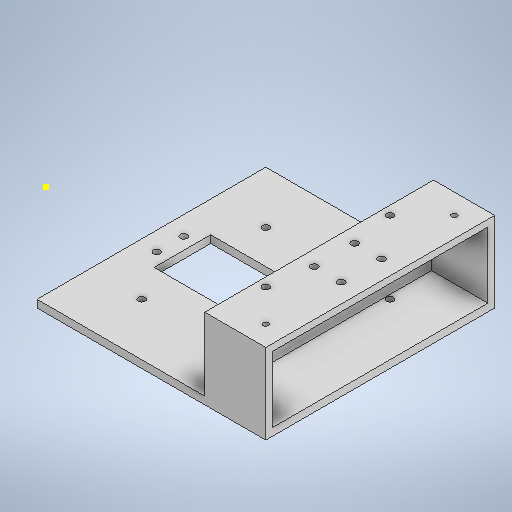
# Autodesk Inventor part: LowerHead
Saved by Autodesk Inventor 2025 (Build 290162000, 162)
## iProperties
Created: 2025-09-02
Part Number: LowerHead
Material: Generic
Document SubType Name: Modeling
Designer: wangb
Density: 1 g/cm^3
Appearance: Default
Author: wangb
Autodesk Inventor part; units mm, degrees
ref_plane "YZ Plane" through (0, 0, 0) normal (1, 0, 0) x (0, 1, 0)
ref_plane "XZ Plane" through (0, 0, 0) normal (0, 1, 0) x (-1, 0, 0)
ref_plane "XY Plane" through (0, 0, 0) normal (0, 0, 1) x (1, 0, 0)
sketch "Sketch1" plane through (0, 0, 0) normal (0, 1, 0) x (-1, 0, 0)
  line L0 (-7.3056, 10.788) -> (-92.3056, 10.788)
  line L1 (-92.3056, 10.788) -> (-92.3056, -74.212)
  line L2 (-92.3056, -74.212) -> (-7.3056, -74.212)
  line L3 (-7.3056, -74.212) -> (-7.3056, 10.788)
  line L4 (-18.8056, -21.212) -> (-59.8056, -21.212)
  line L5 (-59.8056, -21.212) -> (-59.8056, -42.212)
  line L6 (-59.8056, -42.212) -> (-18.8056, -42.212)
  line L7 (-18.8056, -42.212) -> (-18.8056, -21.212)
  circle A0 centre (-14.3056, -26.712) radius 1.3
  circle A1 centre (-14.3056, -36.712) radius 1.3
  circle A2 centre (-64.3056, -26.712) radius 1.3
  circle A3 centre (-64.3056, -36.712) radius 1.3
  circle A4 centre (-75.3056, -39.212) radius 1.3
  circle A5 centre (-85.3056, -39.212) radius 1.3
  circle A6 centre (-75.3056, -24.212) radius 1.3
  circle A7 centre (-85.3052, -24.1286) radius 1.3
  point P0 (0, 0)
  dimension "d0" = 85
  dimension "d1" = 85
  dimension "d2" = 41
  dimension "d3" = 21
  dimension "d4" = 32
  dimension "d5" = 11.5
  dimension "d6" = 2.6
  dimension "d7" = 2.6
  dimension "d8" = 10
  dimension "d9" = 5.5
  dimension "d10" = 5.5
  dimension "d11" = 2.6
  dimension "d12" = 2.6
  dimension "d13" = 10
  dimension "d14" = 5.5
  dimension "d15" = 50
  dimension "d16" = 50
  dimension "d17" = 4.5
  dimension "d31" = 2.6
  dimension "d32" = 2.6
  dimension "d33" = 10
  dimension "d34" = 2.6
  dimension "d35" = 2.6
  dimension "d36" = 10
  dimension "d37" = 15
  dimension "d38" = 35
  dimension "d39" = 17
  dimension "d40" = 17
  constraints: 16 end point, 8 centre point, 4 parallel, 2 horizontal, 2 perpendicular
  measures "d0" distance of L2.end L1.end
  measures "d1" distance of L1.end L0.end
  measures "d2" distance of L6.end L5.end
  measures "d3" distance of L5.end L4.end
  measures "d4" distance between parallel lines of L2 L6
  measures "d5" distance between parallel lines of L3 L7
  measures "d6" diameter of A0
  measures "d7" diameter of A1
  measures "d8" distance of A1.centre A0.centre
  measures "d9" vertical distance of L4.start A0.centre
  measures "d10" vertical distance of L6.end A1.centre
  measures "d11" diameter of A2
  measures "d12" diameter of A3
  measures "d13" distance of A3.centre A2.centre
  measures "d14" vertical distance of L5.end A3.centre
  measures "d15" distance of A2.centre A0.centre
  measures "d16" distance of A3.centre A1.centre
  measures "d17" distance from line of L5 A2.centre
  measures "d31" diameter of A4
  measures "d32" diameter of A5
  measures "d33" distance of A5.centre A4.centre
  measures "d34" diameter of A6
  measures "d35" diameter of A7
  measures "d36" distance of A7.centre A6.centre
  measures "d37" distance of A6.centre A4.centre
  measures "d38" distance from line of L2 A4.centre
  measures "d39" distance from line of A6.centre L1
  measures "d40" distance from line of L1 A4.centre
extrude "Extrusion1" add sketch "Sketch1" along normal blind 2.8 contours L3 L2 L1 L0 | A4 | A5 | A6 | A7
sketch "Sketch2" plane through (0, 2.8, 0) normal (0, 1, 0) x (1, 0, 0)
  line L0 (92.3056, -10.788) -> (92.3056, 74.212) projected
  line L1 (92.3056, 74.212) -> (7.3056, 74.212) projected
  line L2 (7.3056, -10.788) -> (92.3056, -10.788) projected
  point P0 (0, 0)
extrude "Extrusion2" [suppressed]
sketch "Sketch3" plane through (0, 2.8, 0) normal (0, 1, 0) x (1, 0, 0)
  line L0 (7.3056, -10.788) -> (92.3056, -10.788) projected
  line L1 (92.3056, 74.212) -> (7.3056, 74.212) projected
  line L2 (92.3056, -10.788) -> (69.6056, -10.788)
  line L3 (69.6056, -10.788) -> (69.6056, 74.212)
  line L4 (69.6056, 74.212) -> (92.3056, 74.212)
  line L5 (92.3056, 74.212) -> (92.3056, -10.788)
  circle A0 centre (64.3056, 36.712) radius 1.3 projected
  circle A1 centre (75.3056, 24.212) radius 1 projected
  circle A2 centre (75.3056, 24.212) radius 1
  circle A3 centre (75.3056, 39.212) radius 1 projected
  circle A4 centre (75.3056, 39.212) radius 1
  circle A5 centre (85.3056, 39.212) radius 1 projected
  circle A6 centre (85.3056, 39.212) radius 1
  circle A7 centre (85.3056, 24.212) radius 1 projected
  circle A8 centre (85.3056, 24.212) radius 1
  circle A9 centre (84.8056, 66.712) radius 0.95 projected
  circle A10 centre (84.8056, 66.712) radius 1
  circle A11 centre (84.8056, -3.288) radius 0.95 projected
  circle A12 centre (84.8056, -3.288) radius 1
  point P0 (0, 0)
  dimension "d55" = 4
  dimension "d56" = 2
  dimension "d57" = 2
  constraints: 8 end point, 6 centre point, 6 coincident, 2 parallel, 1 horizontal, 1 perpendicular, 1 point on line
  measures "d55" distance edge to line of A0 L3
  measures "d56" diameter of A10
  measures "d57" diameter of A12
extrude "Extrusion3" add sketch "Sketch3" along normal blind 27 contours L3 L1 L5 L0
sketch "Sketch4" plane through (92.3056, 0, 10.788) normal (1, 0, 0) x (0, 0, -1)
  line L0 (85, 2.8) -> (0, 2.8) projected
  line L1 (2.5, 27.3) -> (82.5, 27.3)
  line L2 (82.5, 27.3) -> (82.5, 2.8)
  line L3 (82.5, 2.8) -> (2.5, 2.8)
  line L4 (2.5, 2.8) -> (2.5, 27.3)
  line L5 (0, 0) -> (0, 29.8) projected
  line L6 (85, 0) -> (85, 29.8) projected
  line L7 (0, 0) -> (85, 0) projected
  line L8 (0, 29.8) -> (85, 29.8) projected
  point P0 (10.788, 0)
  point P1 (2.5, 2.8)
  dimension "d60" = 2.5
  dimension "d61" = 2.5
  dimension "d62" = 2.8
  dimension "d63" = 2.5
  constraints: 8 end point, 2 parallel, 1 horizontal, 1 perpendicular, 1 point on line
  measures "d60" distance between parallel lines of L5 L4
  measures "d61" distance between parallel lines of L6 L2
  measures "d62" distance between parallel lines of L7 L0
  measures "d63" distance between parallel lines of L8 L1
extrude "Extrusion4" cut sketch "Sketch4" against normal blind 21 contours L0 L4 L1 L2
sketch "Sketch5" plane through (0, 0, 0) normal (0, -1, 0) x (1, 0, 0)
  circle A0 centre (26.7535, -8.6599) radius 1.3
  circle A1 centre (72.8576, -8.66) radius 1.3
  circle A2 centre (26.7536, -54.764) radius 1.3
  circle A3 centre (72.8576, -54.764) radius 1.3
  line L0 (7.3056, 10.788) -> (92.3056, 10.788) projected
  line L1 (92.3056, 10.788) -> (92.3056, -74.212) projected
  line L2 (7.3056, -74.212) -> (7.3056, 10.788) projected
  line L3 (92.3056, -74.212) -> (7.3056, -74.212) projected
  point P0 (0, 0)
  point P1 (49.2547, -32.4518)
  point P2 (49.2547, -32.4518)
  dimension "d66" = 2.6
  dimension "d67" = 2.6
  dimension "d68" = 2.6
  dimension "d69" = 2.6
  dimension "d70" = 46.1041
  dimension "d71" = 46.1041
  dimension "d72" = 46.1041
  dimension "d73" = 46.1041
  dimension "d74" = 19.448
  dimension "d75" = 19.448
  dimension "d76" = 19.448
  dimension "d77" = 19.448
  constraints: 4 centre point
  measures "d66" diameter of A0
  measures "d67" diameter of A1
  measures "d68" diameter of A2
  measures "d69" diameter of A3
  measures "d70" distance of A1.centre A0.centre
  measures "d71" distance of A2.centre A0.centre
  measures "d72" distance of A3.centre A1.centre
  measures "d73" distance of A3.centre A2.centre
  measures "d74" distance from line of L0 A1.centre
  measures "d75" distance from line of L1 A1.centre
  measures "d76" distance from line of L2 A2.centre
  measures "d77" distance from line of L3 A2.centre
extrude "Extrusion5" cut sketch "Sketch5" against normal blind 100 contours A0 | A1 | A2 | A3
sketch "Sketch6" plane through (0, 29.8, 0) normal (0, 1, 0) x (1, 0, 0)
  point P0 (0, 0)
sketch "Sketch7" plane through (0, 29.8, 0) normal (0, 1, 0) x (1, 0, 0)
  circle A0 centre (75.3056, 39.212) radius 1 projected
  circle A1 centre (75.3056, 39.212) radius 1.3
  circle A2 centre (85.3056, 39.212) radius 1 projected
  circle A3 centre (85.3056, 39.212) radius 1.3
  circle A4 centre (75.3056, 24.212) radius 1 projected
  circle A5 centre (75.3056, 24.212) radius 1.3
  circle A6 centre (85.3056, 24.212) radius 1 projected
  circle A7 centre (85.3056, 24.212) radius 1.3
  point P0 (0, 0)
  dimension "d80" = 2.6
  dimension "d81" = 2.6
  dimension "d82" = 2.6
  dimension "d83" = 2.6
  constraints: 4 centre point, 4 coincident
  measures "d80" diameter of A1
  measures "d81" diameter of A3
  measures "d82" diameter of A5
  measures "d83" diameter of A7
extrude "Extrusion6" cut sketch "Sketch7" against normal blind 10 contours A0 | A1 | A2 | A3 | A4 | A5 | A6 | A7
body "Solid1"
